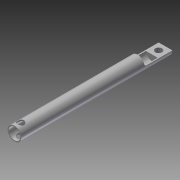
# Autodesk Inventor part: Horizantal Rod
Saved by Autodesk Inventor 2013 (Build 170138000, 138)
## iProperties
Created: 2014-05-22
Part Number: Horizantal Rod
Material: Steel
Document SubType Name: Modeling
Designer: nojessen
Mass: 307.769 g
Surface Area: 387.667 cm^2
Volume: 39.2063 cm^3
Density: 7.85 g/cm^3
Author: nojessen
Autodesk Inventor part; units mm, degrees
ref_plane "YZ Plane" through (0, 0, 0) normal (1, 0, 0) x (0, 1, 0)
ref_plane "XZ Plane" through (0, 0, 0) normal (0, 1, 0) x (-1, 0, 0)
ref_plane "XY Plane" through (0, 0, 0) normal (0, 0, 1) x (1, 0, 0)
sketch "Sketch1" plane through (0, 0, 0) normal (0, 0, 1) x (1, 0, 0)
  circle A0 centre (0, 0) radius 12.7
  circle A1 centre (0, 0) radius 10.795
  line L0 (0, 0) -> (12.7, 0)
  dimension "d0" = 25.4
  dimension "d1" = 21.59
  constraints: 2 coincident, 2 end point, 1 centre point, 1 horizontal, 1 horizontal alignment, 2 other
  measures "d1" diameter of A1
extrude "Extrusion1" add sketch "Sketch1" along normal blind 279.4
ref_plane "Work Plane2" through (0, 12.7, 0) normal (0, 1, 0) x (1, 0, 0)
ref_plane "Work Plane1" through (0, 0, 0) normal (0, 1, 0) x (1, 0, 0)
sketch "Sketch2" plane through (0, 12.7, 0) normal (0, 1, 0) x (1, 0, 0)
  line L0 (0, 0) -> (0, -279.4)
  line L1 (0, -279.4) -> (0, -267.97)
  circle A0 centre (0, -267.97) radius 6.35
  line L2 (0, 0) -> (0, -13.97)
  circle A1 centre (0, -13.97) radius 6.35
  dimension "d6" = 279.4
  dimension "d7" = 11.43
  dimension "d8" = 12.7
  dimension "d9" = 13.97
  dimension "d10" = 12.7
  constraints: 6 end point, 2 centre point, 2 coincident, 2 point on line, 1 vertical
  measures "d6" distance of L0.start L0.end
  measures "d7" distance of L0.end L1.end
  measures "d8" diameter of A0
  measures "d9" distance of L0.start L2.end
  measures "d10" diameter of A1
extrude "Extrusion2" cut sketch "Sketch2" against normal blind 279.4
sketch "Sketch3" plane through (0, 12.7, 0) normal (0, 1, 0) x (1, 0, 0)
  line L0 (0, 0) -> (0, -28.955)
  constraints: 2 end point, 1 vertical
ref_plane "Work Plane4" through (-12.7, 12.7, 0) normal (-1, 0, 0) x (0, 0, 1)
ref_plane "Work Plane3" through (0, 12.7, 0) normal (-1, 0, 0) x (0, 0, 1)
sketch "Sketch4" plane through (-12.7, 12.7, 0) normal (-1, 0, 0) x (0, 0, 1)
  line L0 (0, -12.7) -> (38.1, -12.7)
  line L1 (38.1, -12.7) -> (38.1, 1.5898)
  line L2 (38.1, 1.5898) -> (0, 1.5898)
  line L3 (0, 1.5898) -> (0, -12.7)
  dimension "d15" = 38.1
  constraints: 8 end point, 2 parallel, 1 horizontal, 1 perpendicular
  measures "d15" distance of L2.end L1.end
extrude "Extrusion3" cut sketch "Sketch4" against normal blind 50.8
sketch "Sketch5" plane through (10.795, 0, 38.1) normal (0, 1, 0) x (1, 0, 0)
  line L0 (1.905, 38.1) -> (-23.495, 38.1)
  line L1 (-23.495, 38.1) -> (-23.495, 12.7001)
  line L2 (-23.495, 12.7001) -> (1.905, 12.7001)
  line L3 (1.905, 12.7001) -> (1.905, 38.1)
  point P0 (-10.795, 38.1)
  dimension "d18" = 25.4
  constraints: 8 end point, 2 parallel, 1 horizontal, 1 perpendicular
  measures "d18" distance of L2.end L1.end
extrude "Extrusion4" add sketch "Sketch5" against normal blind 12.7
sketch "Sketch6" plane through (-12.7, 0, 38.1) normal (0, 1, 0) x (1, 0, 0)
  circle A0 centre (12.7, 25.4) radius 6.35
  point P0 (12.7, 38.1)
  dimension "d21" = 12.7
  constraints: 1 centre point
  measures "d21" diameter of A0
extrude "Extrusion5" cut sketch "Sketch6" against normal blind 12.7
sketch "Sketch7" plane through (0, 0, 279.4) normal (0, 0, 1) x (1, 0, 0)
  circle A0 centre (0, 0) radius 12.7 projected
  circle A1 centre (0, 0) radius 44.4632
  constraints: 1 centre point, 1 coincident
extrude "Extrusion6" cut sketch "Sketch7" against normal blind 381
fillet "Fillet1" radius 3.175 2 edges at (-11.7475, 0, 38.1) (11.7475, 0, 38.1)
ref_plane "Work Plane5" through (12.7, 0, 0) normal (-1, 0, 0) x (0, 0, 1)
sketch "Sketch8" plane through (12.7, 0, 0) normal (-1, 0, 0) x (0, 0, 1)
  line L0 (35.1215, 0) -> (51.6315, 0)
  line L1 (51.6315, 0) -> (51.6315, 13.9187)
  line L2 (51.6315, 13.9187) -> (35.1215, 13.9187)
  line L3 (35.1215, 13.9187) -> (35.1215, 0)
  point P0 (0, 0)
  dimension "d28" = 16.51
  constraints: 8 end point, 2 parallel, 1 horizontal, 1 perpendicular
  measures "d28" distance of L2.end L1.end
extrude "Extrusion7" cut sketch "Sketch8" along normal blind 381
fillet "Fillet2" radius 3.175 2 edges at (11.7475, 0, 51.6315) (-11.7475, 0, 51.6315)
body "Solid1"
